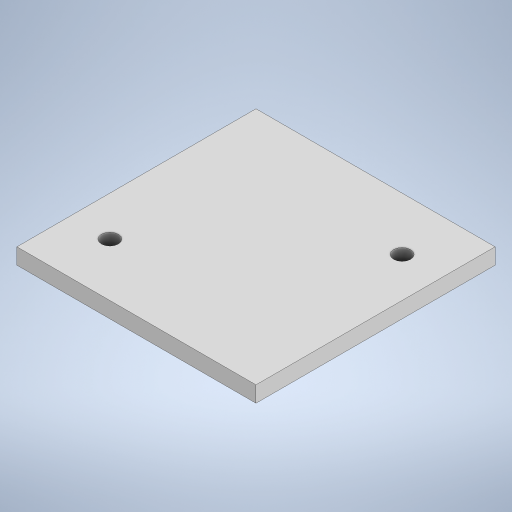
# Autodesk Inventor part: Part2
Saved by Autodesk Inventor 2023 (Build 270158000, 158)
## iProperties
Created: 2022-04-25
Part Number: Part2
Material: 一般
Document SubType Name: Modeling
Designer: yuta
Density: 1 g/cm^3
Appearance: 既定
Author: yuta
Autodesk Inventor part; units mm, degrees
ref_plane "YZ Plane" through (0, 0, 0) normal (1, 0, 0) x (0, 1, 0)
ref_plane "XZ Plane" through (0, 0, 0) normal (0, 1, 0) x (-1, 0, 0)
ref_plane "XY Plane" through (0, 0, 0) normal (0, 0, 1) x (1, 0, 0)
sketch "スケッチ1" plane through (0, 0, 0) normal (0, 1, 0) x (-1, 0, 0)
  line L0 (0, 0) -> (45, 0)
  line L1 (45, 0) -> (45, -45)
  line L2 (45, -45) -> (0, -45)
  line L3 (0, -45) -> (0, 0)
  dimension "d0" = 45
  dimension "d1" = 45
  constraints: 8 end point, 2 parallel, 1 horizontal, 1 perpendicular
  measures "d0" distance of L1.end L2.end
  measures "d1" distance of L0.end L1.end
extrude "押し出し1" add sketch "スケッチ1" along normal blind 3
sketch "スケッチ2" plane through (0, 3, 0) normal (0, 1, 0) x (1, 0, 0)
  line L0 (0, 0) -> (0, 45) projected
  line L1 (0, 45) -> (-45, 45) projected
  line L2 (-45, 45) -> (-45, 0) projected
  line L3 (-45, 0) -> (0, 0) projected
  point P0 (-7.5, 35)
  point P1 (-37.5, 10)
  dimension "d4" = 7.5
  dimension "d5" = 10
  dimension "d6" = 7.5
  dimension "d7" = 10
  measures "d4" distance from line of L0 point (-7.5, 35)
  measures "d5" distance from line of L1 point (-7.5, 35)
  measures "d6" distance from line of L2 point (-37.5, 10)
  measures "d7" distance from line of L3 point (-37.5, 10)
hole "穴1" at (-7.5, 3, -35) at (-37.5, 3, -10) direction (0, -1, 0) diameter 3.2 end through all
